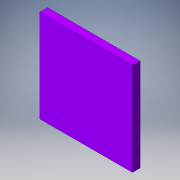
# Autodesk Inventor part: Table_Top
Saved by Autodesk Inventor 2016 (Build 200138000, 138)
## iProperties
Created: 2017-12-15
Part Number: Table_Top
Material: Generic
Document SubType Name: Modeling
Designer: sun01147
Density: 1 g/cm^3
Appearance: Default
Author: sun01147
Autodesk Inventor part; units mm, degrees
ref_plane "YZ Plane" through (0, 0, 0) normal (1, 0, 0) x (0, 1, 0)
ref_plane "XZ Plane" through (0, 0, 0) normal (0, 1, 0) x (-1, 0, 0)
ref_plane "XY Plane" through (0, 0, 0) normal (0, 0, 1) x (1, 0, 0)
sketch "Sketch1" plane through (0, 0, 0) normal (0, 0, 1) x (1, 0, 0)
  line L0 (0, 0) -> (15.24, 0)
  line L1 (0, 0) -> (0, 15.24)
  line L2 (15.24, 0) -> (15.24, 15.24)
  line L3 (0, 15.24) -> (15.24, 15.24)
  dimension "d0" = 15.24
  dimension "d1" = 15.24
  dimension "d2" = 15.24
  constraints: 8 end point, 2 vertical, 1 horizontal
  measures "d0" distance of L0.start L1.end
  measures "d1" distance of L0.start L0.end
  measures "d2" distance of L0.end L2.end
extrude "Extrusion1" add sketch "Sketch1" against normal blind 1.27
body "Solid1"
